Autodesk Fusion 360 part; units mm, degrees
(part 2 of 2)
  spline S324 degree 3 poles (59.345527, 30.078911) (59.290758, 29.007062) (59.056392, 27.951773) (58.746238, 26.920681) knots 0 0 0 0 1 1 1 1
  spline S325 degree 3 poles (58.746238, 26.920681) (57.938054, 24.227361) (56.908234, 21.619384) (55.649784, 19.103124) knots 0 0 0 0 1 1 1 1
  spline S326 degree 3 poles (55.649784, 19.103124) (55.428149, 18.659223) (55.239001, 18.211512) (55.966304, 18.188578) knots 0 0 0 0 1 1 1 1
  spline S327 degree 3 poles (60.056271, 18.18922) (63.158458, 18.207052) (66.260646, 18.256729) (69.361551, 18.232522) knots 0 0 0 0 1 1 1 1
  spline S328 degree 3 poles (69.361551, 18.232522) (70.844834, 18.221046) (70.915521, 18.268177) (70.2691, 19.597325) knots 0 0 0 0 1 1 1 1
  line L64 (57.824695, 31.210622) -> (58.036136, 31.210622)
  line L65 (58.036136, 31.210622) -> (58.723313, 31.210622)
  line L66 (58.723313, 31.210622) -> (61.971978, 31.210622)
  line L67 (61.971978, 31.210622) -> (66.382926, 31.210622)
  line L68 (66.382926, 31.210622) -> (67.629909, 31.210622)
  line L69 (67.629909, 31.210622) -> (68.239393, 31.210622)
  line L70 (68.239393, 31.210622) -> (68.347659, 31.210622)
  spline S329 degree 3 poles (68.347659, 31.210622) (68.362946, 31.212536) (68.376317, 31.216355) (68.390962, 31.21826) knots 0 0 0 0 1 1 1 1
  spline S330 degree 3 poles (68.390962, 31.21826) (69.237357, 31.295322) (69.899706, 32.005424) (69.899706, 32.872207) knots 0 0 0 0 1 1 1 1
  spline S331 degree 3 poles (69.899706, 32.872207) (69.899706, 33.789299) (69.156475, 34.533161) (68.239393, 34.533161) knots 0 0 0 0 1 1 1 1
  line L71 (68.239393, 34.533161) -> (67.238232, 34.533161)
  spline S332 degree 3 poles (67.238232, 34.533161) (67.210847, 34.603849) (67.192373, 34.69302) (67.184094, 34.806378) knots 0 0 0 0 1 1 1 1
  spline S333 degree 3 poles (67.184094, 34.806378) (67.109577, 35.819638) (67.39362, 36.838622) (67.107673, 37.84679) knots 0 0 0 0 1 1 1 1
  line L72 (67.107673, 37.84679) -> (59.124524, 37.84679)
  spline S334 degree 3 poles (59.124524, 37.84679) (58.853853, 37.666553) (58.869781, 37.38251) (58.871685, 37.106747) knots 0 0 0 0 1 1 1 1
  spline S335 degree 3 poles (58.871685, 37.106747) (58.874873, 36.57178) (58.881879, 36.036171) (58.881879, 35.501204) knots 0 0 0 0 1 1 1 1
  spline S336 degree 3 poles (58.881879, 35.501204) (58.881238, 35.124813) (58.883153, 34.778362) (58.709291, 34.53253) knots 0 0 0 0 1 1 1 1
  line L73 (58.709291, 34.53253) -> (57.825958, 34.53253)
  spline S337 degree 3 poles (57.825958, 34.53253) (56.907593, 34.53253) (56.164373, 33.789299) (56.164373, 32.871576) knots 0 0 0 0 1 1 1 1
  spline S338 degree 3 poles (56.164373, 32.871576) (56.164373, 31.953852) (56.905688, 31.210622) (57.824695, 31.210622) knots 0 0 0 0 1 1 1 1
  line L74 (55.966304, 18.188578) -> (59.943585, 18.188578)
  line L75 (62.983152, 18.188578) -> (62.983152, 58.757607)
  line L76 (62.983152, 18.188578) -> (62.983152, 0.48983)
  spline S339 degree 3 poles (59.943585, 18.188578) (59.981148, 18.188812) (60.018709, 18.189027) (60.056271, 18.18922) knots 0.97245282 0.97245282 0.97245282 0.97245282 1 1 1 1
  spline S340 degree 5 poles (71.608432, 3.574986) (71.613145, 3.553029) (71.623752, 3.511309) (71.643206, 3.4553) (71.675256, 3.391951) (71.722096, 3.325335) (71.762896, 3.278211) (71.794751, 3.245199) (71.816511, 3.224158) (71.827521, 3.21388) knots 0 0 0 0 0 0 0.2 0.4 0.6 0.8 1 1 1 1 1 1
  line L77 (71.596739, 3.62947) -> (71.620126, 3.520501)
  spline S341 degree 5 poles (70.551808, 18.350972) (70.552078, 18.326595) (70.555173, 18.280443) (70.567469, 18.219012) (70.597062, 18.150549) (70.648694, 18.079885) (70.697185, 18.030674) (70.736268, 17.99653) (70.76345, 17.974917) (70.777324, 17.964397) knots 0 0 0 0 0 0 0.2 0.4 0.6 0.8 1 1 1 1 1 1
  spline S342 degree 5 poles (71.4091, 15.335391) (71.40249, 15.346502) (71.389231, 15.369114) (71.369226, 15.404203) (71.342303, 15.453494) (71.308032, 15.521324) (71.279808, 15.583695) (71.25796, 15.637325) (71.243043, 15.676611) (71.235497, 15.697138) knots 0 0 0 0 0 0 0.2 0.4 0.6 0.8 1 1 1 1 1 1
  line L78 (70.55116, 18.40932) -> (70.552455, 18.292624)
  line L79 (71.254696, 15.644913) -> (71.216297, 15.749362)
  line L80 (66.521764, 30.848243) -> (66.394816, 31.210622)
  line L81 (67.107673, 37.84679) -> (67.028314, 38.207254)
  spline S343 degree 5 poles (60.241774, 51.061468) (60.241772, 51.061472) (60.241771, 51.061475) (60.241769, 51.061478) (60.241768, 51.061481) (60.241766, 51.061485) knots 0 0 0 0 0 0 0.00000789 0.00000789 0.00000789 0.00000789 0.00000789 0.00000789
  line L82 (60.241767, 51.061483) -> (60.241766, 51.061486)
  line L83 (60.8381, 48.17105) -> (60.758794, 48.335324)
  spline S344 degree 3 poles (61.097336, 47.634071) (61.058101, 47.687058) (61.023561, 47.745941) (60.992478, 47.803593) knots 0.72733862 0.72733862 0.72733862 0.72733862 1 1 1 1
  line L84 (61.705339, 47.91026) -> (59.426231, 52.748691)
  line L85 (61.114396, 47.590593) -> (58.975681, 52.130978)
  line L86 (58.975681, 52.130978) -> (59.426231, 52.748691)
  arc A0 (61.082005, 47.659359) -> (61.705068, 47.910836) centre (61.40066, 47.767447) ccw
  arc A1 (61.632808, 48.011032) -> (61.632808, 48.011032) centre (61.40066, 47.767447) ccw
  spline S345 degree 3 poles (61.603876, 48.075532) (61.676957, 47.906835) (61.811677, 47.675078) (61.641087, 47.532035) knots 0 0 0 0 0.86282034 0.86282034 0.86282034 0.86282034
  spline S346 degree 5 poles (67.035375, 28.406843) (67.020995, 28.241459) (67.010465, 27.900747) (67.049309, 27.359878) (67.19787, 26.589348) (67.509068, 25.585628) (67.846293, 24.783653) (68.15254, 24.198216) (68.382482, 23.817425) (68.503902, 23.629407) knots 0 0 0 0 0 0 0.2 0.4 0.6 0.8 1 1 1 1 1 1
  line L87 (67.070749, 28.813685) -> (67.000001, 28)
  line L88 (68.199998, 24.099999) -> (68.807805, 23.158815)
  constraint horizontal L74
  constraint vertical L75
  constraint perpendicular L39 L76
  constraint parallel L84 L85
  constraint tangent L84 A0
  constraint concentric A0 A1
revolve "Revolve1" add sketch "Bishop" angle 360 about axis through (0, 62.983152, 18.188578) along (0, 0, 1) contours L16 S139 S140 S141 L76 | L16 L37 L76 S342 L79 | S141 S327 S328 L75 L76 S341 | L36 S228 S229 S230 L37 L76 | L36 L39 L76 S340 | S319 S320 L61 S321 L62 S327 S328 L75 S346 | L39 S238 S239 S240 S241 L76 | L61 S321 L62 L67 L68 L75 L80 | S319 S320 S346 | L67 L68 L69 L70 S329 S330 S331 L71 S332 S333 L72 L75 | L35 L72 L75 L81 | S207 S208 S209 S210 S211 S212 S213 L35 S226 S227 L75 picked at (68.331991, 16.452891) picked at (65.733934, 15.576555) picked at (67.707342, 18.050557) picked at (66.366295, 10.192791) picked at (65.858246, 3.454617) picked at (64.40064, 25.205049) picked at (66.67053, 2.30443) picked at (64.379918, 31.089829) picked at (67.197351, 27.040636) picked at (64.383466, 34.621263) picked at (65.706379, 37.966944) picked at (65.265382, 46.82939)
extrude "Extrude2" cut sketch "Bishop" along normal mid plane 24 contours S218 S220 L84 L85 L86 A1 S345 | S344 L85 A0 A1 S345 picked at (60.21943, 50.540033) picked at (61.283905, 47.768826)
extrude "Extrude3" cut sketch "Bishop" along normal mid plane 20 contours S319 S320 S346 picked at (67.197351, 27.040636)
pattern_circular "C-Pattern1" count 6 over 360 about axis through (0, 62.983152, 18.188578) along (0, 0, 1) of "Extrude3"
named bodies: "Bishop"
